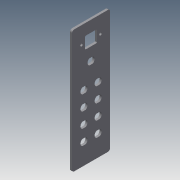
# Autodesk Inventor part: Front-panel
Saved by Autodesk Inventor 2015 SP1 (Build 190203100, 203)
## iProperties
Created: 2015-07-22
Part Number: Front-panel
Material: Generic
Document SubType Name: Modeling
Designer: James
Density: 1 g/cm^3
Appearance: Default
Author: James
Autodesk Inventor part; units mm, degrees
ref_plane "YZ Plane" through (0, 0, 0) normal (1, 0, 0) x (0, 1, 0)
ref_plane "XZ Plane" through (0, 0, 0) normal (0, 1, 0) x (-1, 0, 0)
ref_plane "XY Plane" through (0, 0, 0) normal (0, 0, 1) x (1, 0, 0)
sketch "Sketch1" plane through (0, 0, 0) normal (1, 0, 0) x (0, 1, 0)
  line L0 (25.0568, 85.4307) -> (-25.9432, 85.4307)
  line L1 (-25.9432, 85.4307) -> (-25.9432, -79.5693)
  line L2 (-25.9432, -79.5693) -> (25.0568, -79.5693)
  line L3 (25.0568, -79.5693) -> (25.0568, 85.4307)
  point P0 (0, 0)
  dimension "d0" = 165
  dimension "d1" = 51
  constraints: 8 end point, 2 parallel, 1 horizontal, 1 perpendicular
  measures "d0" distance between parallel lines of L0 L2
  measures "d1" distance between parallel lines of L3 L1
extrude "Extrusion1" add sketch "Sketch1" along normal blind 3
fillet "Fillet1" radius 3 4 edges at (1.5, 25.0568, 85.4307) (1.5, -25.9432, 85.4307) (1.5, 25.0568, -79.5693) (1.5, -25.9432, -79.5693)
sketch "Sketch2" plane through (3, 0, 0) normal (1, 0, 0) x (0, 0, -1)
  line L0 (-77.4307, 22.0568) -> (71.5693, 22.0568)
  line L1 (71.5693, 22.0568) -> (71.5693, -22.9432)
  line L2 (71.5693, -22.9432) -> (-77.4307, -22.9432)
  line L3 (-77.4307, -22.9432) -> (-77.4307, 22.0568)
  line L4 (-85.4307, 22.0568) -> (-85.4307, -22.9432) projected
  line L5 (79.5693, -22.9432) -> (79.5693, 22.0568) projected
  line L6 (-82.4307, -25.9432) -> (76.5693, -25.9432) projected
  line L7 (76.5693, 25.0568) -> (-82.4307, 25.0568) projected
  point P0 (0, 0)
  dimension "d5" = 149
  dimension "d6" = 45
  dimension "d9" = 165
  dimension "d10" = 8
  dimension "d11" = 51
  dimension "d12" = 3
  constraints: 8 end point, 2 parallel, 1 horizontal, 1 perpendicular
  measures "d5" distance between parallel lines of L3 L1
  measures "d6" distance between parallel lines of L2 L0
  measures "d9" distance between parallel lines of L4 L5
  measures "d10" distance between parallel lines of L5 L1
  measures "d11" distance between parallel lines of L6 L7
  measures "d12" distance between parallel lines of L7 L0
extrude "Extrusion2" cut sketch "Sketch2" against normal blind 0.1
sketch "Sketch4" plane through (2.9, 0, 0) normal (1, 0, 0) x (0, 0, -1)
  line L0 (-77.4307, 22.0568) -> (71.5693, 22.0568)
  line L1 (71.5693, 22.0568) -> (71.5693, -22.9432)
  line L2 (71.5693, -22.9432) -> (-77.4307, -22.9432)
  line L3 (-77.4307, -22.9432) -> (-77.4307, 22.0568)
  line L4 (-41.5807, 1.8676) -> (-33.2807, 1.8676)
  line L5 (-33.2807, 1.8676) -> (-33.2807, -2.7541)
  line L6 (-33.2807, -2.7541) -> (-41.5807, -2.7541)
  line L7 (-41.5807, -2.7541) -> (-41.5807, 1.8676)
  line L8 (-41.5807, 1.8676) -> (-33.2807, -2.7541) construction
  line L9 (-33.2807, 1.8676) -> (-41.5807, -2.7541) construction
  arc A0 (-33.2807, 1.8676) -> (-41.5807, 1.8676) centre (-37.4307, -0.4432) ccw
  line L10 (-12.5807, 6.7459) -> (-4.2807, 6.7459)
  line L11 (-4.2807, 6.7459) -> (-4.2807, 11.3676)
  line L12 (-4.2807, 11.3676) -> (-12.5807, 11.3676)
  line L13 (-12.5807, 11.3676) -> (-12.5807, 6.7459)
  line L14 (-12.5807, 6.7459) -> (-4.2807, 11.3676) construction
  line L15 (-4.2807, 6.7459) -> (-12.5807, 11.3676) construction
  arc A1 (-4.2807, 11.3676) -> (-12.5807, 11.3676) centre (-8.4307, 9.0568) ccw
  arc A2 (-12.5807, 6.7459) -> (-4.2807, 6.7459) centre (-8.4307, 9.0568) ccw
  line L16 (7.4193, 11.3676) -> (15.7193, 11.3676)
  line L17 (15.7193, 11.3676) -> (15.7193, 6.7459)
  line L18 (15.7193, 6.7459) -> (7.4193, 6.7459)
  line L19 (7.4193, 6.7459) -> (7.4193, 11.3676)
  line L20 (7.4193, 11.3676) -> (15.7193, 6.7459) construction
  line L21 (15.7193, 11.3676) -> (7.4193, 6.7459) construction
  arc A3 (15.7193, 11.3676) -> (7.4193, 11.3676) centre (11.5693, 9.0568) ccw
  arc A4 (7.4193, 6.7459) -> (15.7193, 6.7459) centre (11.5693, 9.0568) ccw
  line L22 (27.4193, 6.7459) -> (35.7193, 6.7459)
  line L23 (35.7193, 6.7459) -> (35.7193, 11.3676)
  line L24 (35.7193, 11.3676) -> (27.4193, 11.3676)
  line L25 (27.4193, 11.3676) -> (27.4193, 6.7459)
  line L26 (27.4193, 6.7459) -> (35.7193, 11.3676) construction
  line L27 (35.7193, 6.7459) -> (27.4193, 11.3676) construction
  line L28 (55.7193, -12.2541) -> (47.4193, -12.2541)
  line L29 (47.4193, -12.2541) -> (47.4193, -7.6324)
  line L30 (47.4193, -7.6324) -> (55.7193, -7.6324)
  line L31 (55.7193, -7.6324) -> (55.7193, -12.2541)
  line L32 (55.7193, -12.2541) -> (47.4193, -7.6324) construction
  line L33 (47.4193, -12.2541) -> (55.7193, -7.6324) construction
  line L34 (27.4193, -12.2541) -> (35.7193, -12.2541)
  line L35 (35.7193, -12.2541) -> (35.7193, -7.6324)
  line L36 (35.7193, -7.6324) -> (27.4193, -7.6324)
  line L37 (27.4193, -7.6324) -> (27.4193, -12.2541)
  line L38 (27.4193, -12.2541) -> (35.7193, -7.6324) construction
  line L39 (35.7193, -12.2541) -> (27.4193, -7.6324) construction
  line L40 (15.7193, -12.2541) -> (7.4193, -12.2541)
  line L41 (7.4193, -12.2541) -> (7.4193, -7.6324)
  line L42 (7.4193, -7.6324) -> (15.7193, -7.6324)
  line L43 (15.7193, -7.6324) -> (15.7193, -12.2541)
  line L44 (15.7193, -12.2541) -> (7.4193, -7.6324) construction
  line L45 (7.4193, -12.2541) -> (15.7193, -7.6324) construction
  line L46 (-12.5807, -12.2541) -> (-4.2807, -12.2541)
  line L47 (-4.2807, -12.2541) -> (-4.2807, -7.6324)
  line L48 (-4.2807, -7.6324) -> (-12.5807, -7.6324)
  line L49 (-12.5807, -7.6324) -> (-12.5807, -12.2541)
  line L50 (-12.5807, -12.2541) -> (-4.2807, -7.6324) construction
  line L51 (-4.2807, -12.2541) -> (-12.5807, -7.6324) construction
  arc A5 (-4.2807, -7.6324) -> (-12.5807, -7.6324) centre (-8.4307, -9.9432) ccw
  arc A6 (-12.5807, -12.2541) -> (-4.2807, -12.2541) centre (-8.4307, -9.9432) ccw
  arc A7 (15.7193, -7.6324) -> (7.4193, -7.6324) centre (11.5693, -9.9432) ccw
  arc A8 (7.4193, -12.2541) -> (15.7193, -12.2541) centre (11.5693, -9.9432) ccw
  arc A9 (35.7193, -7.6324) -> (27.4193, -7.6324) centre (31.5693, -9.9432) ccw
  arc A10 (27.4193, -12.2541) -> (35.7193, -12.2541) centre (31.5693, -9.9432) ccw
  arc A11 (55.7193, -7.6324) -> (47.4193, -7.6324) centre (51.5693, -9.9432) ccw
  arc A12 (47.4193, -12.2541) -> (55.7193, -12.2541) centre (51.5693, -9.9432) ccw
  arc A13 (35.7193, 11.3676) -> (27.4193, 11.3676) centre (31.5693, 9.0568) ccw
  arc A14 (27.4193, 6.7459) -> (35.7193, 6.7459) centre (31.5693, 9.0568) ccw
  line L52 (55.7193, 6.7459) -> (47.4193, 6.7459)
  line L53 (47.4193, 6.7459) -> (47.4193, 11.3676)
  line L54 (47.4193, 11.3676) -> (55.7193, 11.3676)
  line L55 (55.7193, 11.3676) -> (55.7193, 6.7459)
  line L56 (55.7193, 6.7459) -> (47.4193, 11.3676) construction
  line L57 (47.4193, 6.7459) -> (55.7193, 11.3676) construction
  arc A15 (55.7193, 11.3676) -> (47.4193, 11.3676) centre (51.5693, 9.0568) ccw
  arc A16 (47.4193, 6.7459) -> (55.7193, 6.7459) centre (51.5693, 9.0568) ccw
  arc A17 (-41.5807, -2.7541) -> (-33.2807, -2.7541) centre (-37.4307, -0.4432) ccw
  line L58 (-70.4307, -8.4432) -> (-70.4307, 7.5568)
  line L59 (-70.4307, 7.5568) -> (-54.4307, 7.5568)
  line L60 (-54.4307, 7.5568) -> (-54.4307, -8.4432)
  line L61 (-54.4307, -8.4432) -> (-70.4307, -8.4432)
  line L62 (-70.4307, -8.4432) -> (-54.4307, 7.5568) construction
  line L63 (-70.4307, 7.5568) -> (-54.4307, -8.4432) construction
  point P0 (0, 0)
  point P1 (-62.4307, -0.4432)
  point P2 (-62.4307, -13.1432)
  point P3 (-62.4307, 12.2568)
  dimension "d16" = 20
  dimension "d17" = 20
  dimension "d18" = 20
  dimension "d20" = 19
  dimension "d25" = 20
  dimension "d26" = 20
  dimension "d27" = 20
  dimension "d28" = 19
  dimension "d29" = 19
  dimension "d43" = 13
  dimension "d44" = 45
  dimension "d45" = 13
  dimension "d46" = 13
  dimension "d47" = 13
  dimension "d70" = 22.5
  dimension "d71" = 8.3
  dimension "d72" = 4.75
  dimension "d73" = 40
  dimension "d74" = 20.1892
  dimension "d75" = 8.3
  dimension "d76" = 4.75
  dimension "d77" = 8.3
  dimension "d78" = 4.75
  dimension "d79" = 8.3
  dimension "d81" = 8.3
  dimension "d82" = 8.3
  dimension "d83" = 8.3
  dimension "d84" = 8.3
  dimension "d85" = 4.75
  dimension "d86" = 4.75
  dimension "d88" = 4.75
  dimension "d90" = 4.75
  dimension "d98" = 20
  dimension "d100" = 20
  dimension "d101" = 8.3
  dimension "d104" = 16
  dimension "d105" = 16
  dimension "d106" = 15
  dimension "d107" = 22.5
  dimension "d108" = 8
  dimension "d109" = 8
  dimension "d110" = 12.7
  dimension "d111" = 12.7
  constraints: 128 end point, 36 point on circle, 24 midpoint, 22 parallel, 18 centre point, 15 coincident, 11 perpendicular, 10 horizontal, 1 vertical
  measures "d16" distance of point (51.569, 9.057) point (31.569, 9.057)
  measures "d17" distance of point (11.569, 9.057) point (31.569, 9.057)
  measures "d18" distance of point (11.569, 9.057) point (-8.431, 9.057)
  measures "d20" distance of point (-8.431, 9.057) point (-8.431, -9.943)
  measures "d25" distance of point (51.569, -9.943) point (31.569, -9.943)
  measures "d26" distance of point (11.569, -9.943) point (31.569, -9.943)
  measures "d27" distance of point (-8.431, -9.943) point (11.569, -9.943)
  measures "d28" distance of point (11.569, -9.943) point (11.569, 9.057)
  measures "d29" distance of point (31.569, 9.057) point (31.569, -9.943)
  measures "d43" distance from line of point (-8.431, -9.943) L2
  measures "d44" distance of L2.end L0.start
  measures "d45" distance from line of L2 point (11.569, -9.943)
  measures "d46" distance from line of L2 point (31.569, -9.943)
  measures "d47" distance from line of L2 point (51.569, -9.943)
  measures "d70" distance from line of point (-37.431, -0.443) L0
  measures "d71" distance between parallel lines of L5 L7
  measures "d72" radius of A0
  measures "d73" distance from line of A0.centre L3
  measures "d74" distance between parallel lines of L0 L4
  measures "d75" distance between parallel lines of L11 L13
  measures "d76" radius of A2
  measures "d77" distance between parallel lines of L19 L17
  measures "d78" radius of A3
  measures "d79" distance between parallel lines of L25 L23
  measures "d81" distance between parallel lines of L31 L29
  measures "d82" distance between parallel lines of L37 L35
  measures "d83" distance between parallel lines of L43 L41
  measures "d84" distance between parallel lines of L47 L49
  measures "d85" radius of A6
  measures "d86" radius of A7
  measures "d88" radius of A10
  measures "d90" radius of A13
  measures "d98" distance from line of L1 A11.centre
  measures "d100" distance from line of L1 point (51.569, 9.057)
  measures "d101" distance between parallel lines of L55 L53
  measures "d104" distance between parallel lines of L60 L58
  measures "d105" distance between parallel lines of L61 L59
  measures "d106" distance from line of point (-62.431, -0.443) L3
  measures "d107" distance from line of point (-62.431, -0.443) L2
  measures "d108" distance from line of point (-62.431, 12.257) L60
  measures "d109" distance from line of L60 point (-62.431, -13.143)
  measures "d110" distance of point (-62.431, -0.443) point (-62.431, -13.143)
  measures "d111" distance of point (-62.431, 12.257) point (-62.431, -0.443)
extrude "Extrusion3" cut sketch "Sketch4" against normal blind 20 contours A0 L4 | L4 L5 L6 L7 | L6 A17 | L13 L12 L11 L10 | L10 A2 | A1 L12 | A3 L16 | L16 L17 L18 L19 | L18 A4 | L25 L24 L23 L22 | L22 A14 | A13 L24 | A12 L28 | L28 L29 L30 L31 | L30 A11 | L37 L36 L35 L34 | L34 A10 | A9 L36 | A8 L40 | L40 L41 L42 L43 | L42 A7 | L49 L48 L47 L46 | L46 A6 | A5 L48 | A16 L52 | L52 L53 L54 L55 | L54 A15 | L58 L59 L60 L61
fillet "Fillet2" radius 1 4 edges at (1.45, 7.5568, 54.4307) (1.45, -8.4432, 54.4307) (1.45, -8.4432, 70.4307) (1.45, 7.5568, 70.4307)
hole "Hole4" at (2.9, -0.4432, 37.4307) at (2.9, 9.0568, -11.5693) at (2.9, 9.0568, 8.4307) at (2.9, 9.0568, -31.5693) at (2.9, 9.0568, -51.5693) at (2.9, -9.9432, 8.4307) at (2.9, -9.9432, -11.5693) at (2.9, -9.9432, -31.5693) at (2.9, -9.9432, -51.5693) at (2.9, -13.1432, 62.4307) at (2.9, 12.2568, 62.4307) direction (-1, 0, 0) diameter 3.4 end through all clearance for "Flat Head Machine Screw" size "M3" standard "Ansi Metric M Profile"
sketch "Sketch9" plane through (3, 0, 0) normal (1, 0, 0) x (0, 0, -1)
  line L0 (-77.4307, -22.9432) -> (-77.4307, 22.0568) projected
  line L1 (-77.4307, 22.0568) -> (71.5693, 22.0568) projected
  line L2 (71.5693, 22.0568) -> (71.5693, -22.9432) projected
  line L3 (71.5693, -22.9432) -> (-77.4307, -22.9432) projected
  arc A0 (76.5693, -25.9432) -> (79.5693, -22.9432) centre (76.5693, -22.9432) ccw projected
  line L4 (79.5693, -22.9432) -> (79.5693, 22.0568) projected
  arc A1 (79.5693, 22.0568) -> (76.5693, 25.0568) centre (76.5693, 22.0568) ccw projected
  line L5 (76.5693, 25.0568) -> (-82.4307, 25.0568) projected
  arc A2 (-82.4307, 25.0568) -> (-85.4307, 22.0568) centre (-82.4307, 22.0568) ccw projected
  line L6 (-85.4307, 22.0568) -> (-85.4307, -22.9432) projected
  arc A3 (-85.4307, -22.9432) -> (-82.4307, -25.9432) centre (-82.4307, -22.9432) ccw projected
  line L7 (-82.4307, -25.9432) -> (76.5693, -25.9432) projected
  point P0 (0, 0)
extrude "Extrusion4" cut sketch "Sketch9" against normal blind 0.1
equation "\"d10\" = -0.5 * d5 + 0.5 * d9"
equation "\"d12\" = -0.5 * d6 + 0.5 * d11"
equation "\"d25\" = d16"
equation "\"d26\" = d17"
equation "\"d27\" = d18"
equation "\"d28\" = d20"
equation "\"d29\" = d28"
equation "\"d43\" = -0.5 * d20 + 0.5 * d44"
equation "\"d45\" = d43"
equation "\"d46\" = d45"
equation "\"d47\" = d46"
equation "\"d78\" = d76"
equation "\"d85\" = d76"
equation "\"d86\" = d85"
equation "\"d88\" = d86"
equation "\"d90\" = d78"
body "Solid1"
